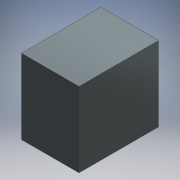
# Autodesk Inventor part: Left leg
Saved by Autodesk Inventor 2016 (Build 200138000, 138)
## iProperties
Created: 2017-05-09
Part Number: Left leg
Material: Iron, Cast
Document SubType Name: Modeling
Designer: M220404
Density: 7.15 g/cm^3
Appearance: Iron Gray
Author: M220404
Autodesk Inventor part; units mm, degrees
ref_plane "YZ Plane" through (0, 0, 0) normal (1, 0, 0) x (0, 1, 0)
ref_plane "XZ Plane" through (0, 0, 0) normal (0, 1, 0) x (-1, 0, 0)
ref_plane "XY Plane" through (0, 0, 0) normal (0, 0, 1) x (1, 0, 0)
sketch "Sketch1" plane through (0, 0, 0) normal (0, 1, 0) x (-1, 0, 0)
  line L0 (0, 0) -> (-422, 0)
  line L1 (-422, 0) -> (-422, -548)
  line L2 (-422, -548) -> (0, -548)
  line L3 (0, -548) -> (0, 0)
  line L4 (-23, -23) -> (-399, -23)
  line L5 (-399, -23) -> (-399, -525)
  line L6 (-399, -525) -> (-23, -525)
  line L7 (-23, -525) -> (-23, -23)
  dimension "d0" = 422
  dimension "d1" = 548
  dimension "d4" = 23
  constraints: 16 end point, 4 parallel, 2 perpendicular, 1 horizontal, 3 other
  measures "d0" distance of L2.end L1.end
  measures "d1" distance of L1.end L0.end
  measures "d4" distance between parallel lines of L3 L7
extrude "Extrusion2" add sketch "Sketch1" along normal blind 583
sketch "Sketch2" plane through (422, 0, -548) normal (0, 0, -1) x (-1, 0, 0)
  line L0 (88, 495) -> (298, 495)
  line L1 (298, 495) -> (298, 150)
  line L2 (298, 150) -> (88, 150)
  line L3 (88, 150) -> (88, 495)
  line L4 (0, 583) -> (422, 583) projected
  line L5 (422, 0) -> (422, 583) projected
  line L6 (0, 0) -> (0, 583) projected
  dimension "d7" = 210
  dimension "d8" = 345
  dimension "d9" = 88
  dimension "d11" = 88
  constraints: 8 end point, 2 parallel, 1 horizontal, 1 perpendicular
  measures "d7" distance of L1.end L2.end
  measures "d8" distance of L0.end L1.end
  measures "d9" distance between parallel lines of L4 L0
  measures "d11" distance between parallel lines of L6 L3
extrude "Extrusion3" cut sketch "Sketch2" against normal up to next
sketch "Sketch3" plane through (0, 583, 0) normal (0, 1, 0) x (1, 0, 0)
  line L0 (399, 23) -> (23, 23) projected
  line L1 (23, 525) -> (399, 525) projected
  line L2 (202, 23) -> (127, 23)
  line L3 (127, 23) -> (127, 525)
  line L4 (127, 525) -> (202, 525)
  line L5 (202, 525) -> (202, 23)
  line L6 (23, 23) -> (23, 525) projected
  point P0 (0, 0)
  dimension "d14" = 75
  dimension "d15" = 104
  constraints: 8 end point, 2 parallel, 2 point on line, 1 horizontal, 1 perpendicular
  measures "d14" distance between parallel lines of L3 L5
  measures "d15" distance between parallel lines of L3 L6
extrude "Extrusion4" add sketch "Sketch3" against normal up to surface (88 mm away) contours L0 L3 L1 L5
sketch "Sketch4" plane through (0, 583, 0) normal (0, 1, 0) x (1, 0, 0)
  line L0 (399, 23) -> (202, 23) projected
  line L1 (202, 525) -> (334, 525) projected
  line L2 (399, 23) -> (345, 23)
  line L3 (345, 23) -> (345, 525)
  line L4 (345, 525) -> (399, 525)
  line L5 (399, 525) -> (399, 23)
  point P0 (0, 0)
  dimension "d18" = 54
  constraints: 8 end point, 2 parallel, 1 horizontal, 1 perpendicular, 1 point on line
  measures "d18" distance between parallel lines of L3 L5
extrude "Extrusion5" add sketch "Sketch4" against normal up to surface (88 mm away)
sketch "Sketch5" plane through (0, 583, 0) normal (0, 1, 0) x (1, 0, 0)
  circle A0 centre (377, 378) radius 8
  circle A1 centre (377, 200) radius 8
  line L0 (422, 548) -> (0, 548) projected
  line L1 (0, 0) -> (422, 0) projected
  line L2 (422, 0) -> (422, 548) projected
  circle A2 centre (157, 200) radius 8
  circle A3 centre (157, 378) radius 8
  line L3 (202, 525) -> (202, 23) projected
  dimension "d21" = 16
  dimension "d22" = 16
  dimension "d23" = 170
  dimension "d24" = 200
  dimension "d25" = 45
  dimension "d26" = 45
  dimension "d27" = 170
  dimension "d28" = 200
  dimension "d29" = 16
  dimension "d30" = 16
  dimension "d31" = 45
  dimension "d32" = 45
  constraints: 4 centre point
  measures "d21" diameter of A1
  measures "d22" diameter of A0
  measures "d23" distance from line of L0 A0.centre
  measures "d24" distance from line of L1 A1.centre
  measures "d25" distance from line of L2 A1.centre
  measures "d26" distance from line of L2 A0.centre
  measures "d27" distance from line of L0 A3.centre
  measures "d28" distance from line of L1 A2.centre
  measures "d29" diameter of A2
  measures "d30" diameter of A3
  measures "d31" distance from line of L3 A2.centre
  measures "d32" distance from line of L3 A3.centre
extrude "Extrusion6" cut sketch "Sketch5" against normal blind 16
sketch "Sketch6" plane through (0, 0, 0) normal (0, -1, 0) x (1, 0, 0)
  line L0 (399, -525) -> (345, -525) projected
  line L1 (23, -23) -> (23, -525) projected
  line L2 (399, -525) -> (23, -525)
  line L3 (23, -525) -> (23, -23)
  line L4 (23, -23) -> (399, -23)
  line L5 (399, -23) -> (399, -525)
  point P0 (0, 0)
  constraints: 8 end point, 2 parallel, 1 horizontal, 1 perpendicular
extrude "Extrusion7" add sketch "Sketch6" against normal blind 123
body "Solid2"
